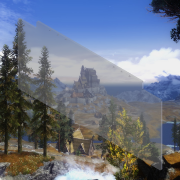
# Autodesk Inventor part: C17_TK_VerticalElectricBoard
Saved by Autodesk Inventor 2015 SP1 (Build 190203100, 203)
## iProperties
Created: 2016-01-21
Part Number: C17_TK_VerticalElectricBoard
Material: Polycarbonate, Clear
Document SubType Name: Modeling
Designer: TheeTimatahee
Density: 1.2 g/cm^3
Appearance: Polycarbonate - Clear
Mass: 547.475 g
Surface Area: 1990.05 cm^2
Volume: 456.229 cm^3
Author: TheeTimatahee
Autodesk Inventor part; units mm, degrees
ref_plane "YZ Plane" through (0, 0, 0) normal (1, 0, 0) x (0, 1, 0)
ref_plane "XZ Plane" through (0, 0, 0) normal (0, 1, 0) x (-1, 0, 0)
ref_plane "XY Plane" through (0, 0, 0) normal (0, 0, 1) x (1, 0, 0)
sketch "Sketch1" plane through (0, 0, 0) normal (0, 0, 1) x (1, 0, 0)
  line L0 (-228.6, -107.95) -> (228.6, -107.95)
  line L1 (168.402, 107.95) -> (-168.402, 107.95)
  line L2 (-171.577, 91.059) -> (-171.577, 109.9058) projected
  line L3 (-171.577, 91.059) -> (-173.736, 88.9) projected
  line L4 (-232.664, 88.9) -> (-173.736, 88.9) projected
  line L5 (-232.664, 88.9) -> (-234.823, 91.059) projected
  line L6 (-234.823, 109.9058) -> (-234.823, 91.059) projected
  line L7 (-171.577, 109.9058) -> (-234.823, 109.9058) projected
  circle A0 centre (-177.8, 101.6) radius 2.0701 projected
  circle A1 centre (-190.5, 101.6) radius 2.0701 projected
  circle A2 centre (-203.2, 101.6) radius 2.0701 projected
  circle A3 centre (-215.9, 101.6) radius 2.0701 projected
  circle A4 centre (-228.6, 101.6) radius 2.0701 projected
  line L8 (234.823, 109.9058) -> (234.823, 91.059) projected
  line L9 (234.823, 91.059) -> (232.664, 88.9) projected
  line L10 (173.736, 88.9) -> (232.664, 88.9) projected
  line L11 (173.736, 88.9) -> (171.577, 91.059) projected
  line L12 (171.577, 109.9058) -> (171.577, 91.059) projected
  line L13 (234.823, 109.9058) -> (171.577, 109.9058) projected
  circle A5 centre (177.8, 101.6) radius 2.0701 projected
  circle A6 centre (190.5, 101.6) radius 2.0701 projected
  circle A7 centre (203.2, 101.6) radius 2.0701 projected
  circle A8 centre (215.9, 101.6) radius 2.0701 projected
  circle A9 centre (228.6, 101.6) radius 2.0701 projected
  line L14 (168.402, 107.95) -> (168.402, 85.725)
  line L15 (168.402, 85.725) -> (228.6, 85.725)
  line L16 (-168.402, 107.95) -> (-168.402, 85.725)
  line L17 (-168.402, 85.725) -> (-228.6, 85.725)
  line L18 (-228.6, 85.725) -> (-228.6, -107.95)
  line L19 (228.6, -107.95) -> (228.6, 85.725)
  point P0 (0, 0)
  dimension "d4" = 3.175
  dimension "d5" = 3.175
  dimension "d6" = 3.175
  dimension "d7" = 3.175
  dimension "d8" = 457.2
  dimension "d9" = 215.9
  constraints: 16 end point, 2 parallel, 1 horizontal, 1 perpendicular
  measures "d4" distance between parallel lines of L10 L15
  measures "d5" distance between parallel lines of L12 L14
  measures "d6" distance between parallel lines of L4 L17
  measures "d7" distance between parallel lines of L16 L2
  measures "d8" distance of L0.start L0.end
  measures "d9" distance between parallel lines of L1 L0
extrude "Extrusion1" add sketch "Sketch1" along normal blind 4.7625 contours L18 L17 L16 L1 L14 L15 L19 L0
fillet "Fillet1" radius 3.175 8 edges at (228.6, -107.95, 2.3813) (168.402, 107.95, 2.3813) (168.402, 85.725, 2.3813) (228.6, 85.725, 2.3813) (-168.402, 107.95, 2.3813) (-168.402, 85.725, 2.3813) (-228.6, 85.725, 2.3813) (-228.6, -107.95, 2.3813)
sketch "Sketch2" plane through (0, 0, 0) normal (0, 0, -1) x (-1, 0, 0)
  arc A0 (103.6687, -25.2476) -> (99.5313, -25.2476) centre (101.6, -25.3238) ccw projected
  line L0 (78.2687, -25.2476) -> (99.5313, -25.2476) projected
  arc A1 (78.2687, -25.2476) -> (74.1313, -25.2476) centre (76.2, -25.3238) ccw projected
  line L1 (52.8687, -25.2476) -> (74.1313, -25.2476) projected
  arc A2 (52.8687, -25.2476) -> (48.7313, -25.2476) centre (50.8, -25.3238) ccw projected
  line L2 (27.4687, -25.2476) -> (48.7313, -25.2476) projected
  arc A3 (27.4687, -25.2476) -> (23.3313, -25.2476) centre (25.4, -25.3238) ccw projected
  line L3 (2.0687, -25.2476) -> (23.3313, -25.2476) projected
  arc A4 (2.0687, -25.2476) -> (-2.0687, -25.2476) centre (0, -25.3238) ccw projected
  line L4 (-23.3313, -25.2476) -> (-2.0687, -25.2476) projected
  arc A5 (-23.3313, -25.2476) -> (-27.4687, -25.2476) centre (-25.4, -25.3238) ccw projected
  line L5 (-48.7313, -25.2476) -> (-27.4687, -25.2476) projected
  arc A6 (-48.7313, -25.2476) -> (-52.8687, -25.2476) centre (-50.8, -25.3238) ccw projected
  line L6 (-74.1313, -25.2476) -> (-52.8687, -25.2476) projected
  arc A7 (-74.1313, -25.2476) -> (-78.2687, -25.2476) centre (-76.2, -25.3238) ccw projected
  line L7 (-99.5313, -25.2476) -> (-78.2687, -25.2476) projected
  arc A8 (-99.5313, -25.2476) -> (-103.6687, -25.2476) centre (-101.6, -25.3238) ccw projected
  line L8 (-124.9313, -25.2476) -> (-103.6687, -25.2476) projected
  arc A9 (-124.9313, -25.2476) -> (-129.0687, -25.2476) centre (-127, -25.3238) ccw projected
  line L9 (-355.6, -25.2476) -> (-129.0687, -25.2476) projected
  line L10 (-355.6, -12.6238) -> (-355.6, -25.2476) projected
  line L11 (355.6, -12.6238) -> (-355.6, -12.6238) projected
  line L12 (355.6, -25.2476) -> (355.6, -12.6238) projected
  line L13 (129.0687, -25.2476) -> (355.6, -25.2476) projected
  arc A10 (129.0687, -25.2476) -> (124.9313, -25.2476) centre (127, -25.3238) ccw projected
  line L14 (103.6687, -25.2476) -> (124.9313, -25.2476) projected
  arc A11 (-99.5313, 101.7524) -> (-103.6687, 101.7524) centre (-101.6, 101.6762) ccw projected
  line L15 (-124.9313, 101.7524) -> (-103.6687, 101.7524) projected
  arc A12 (-124.9313, 101.7524) -> (-129.0687, 101.7524) centre (-127, 101.6762) ccw projected
  line L16 (-175.7355, 101.7524) -> (-129.0687, 101.7524) projected
  arc A13 (-175.7355, 101.7524) -> (-179.8645, 101.7524) centre (-177.8, 101.6) ccw projected
  line L17 (-188.4355, 101.7524) -> (-179.8645, 101.7524) projected
  arc A14 (-188.4355, 101.7524) -> (-192.5645, 101.7524) centre (-190.5, 101.6) ccw projected
  line L18 (-201.1355, 101.7524) -> (-192.5645, 101.7524) projected
  arc A15 (-201.1355, 101.7524) -> (-205.2645, 101.7524) centre (-203.2, 101.6) ccw projected
  line L19 (-213.8355, 101.7524) -> (-205.2645, 101.7524) projected
  arc A16 (-213.8355, 101.7524) -> (-217.9645, 101.7524) centre (-215.9, 101.6) ccw projected
  line L20 (-226.5355, 101.7524) -> (-217.9645, 101.7524) projected
  arc A17 (-226.5355, 101.7524) -> (-230.6645, 101.7524) centre (-228.6, 101.6) ccw projected
  line L21 (-355.6, 101.7524) -> (-230.6645, 101.7524) projected
  line L22 (-355.6, 114.3) -> (-355.6, 101.7524) projected
  line L23 (355.6, 114.3) -> (-355.6, 114.3) projected
  line L24 (355.6, 101.7524) -> (355.6, 114.3) projected
  line L25 (230.6645, 101.7524) -> (355.6, 101.7524) projected
  arc A18 (230.6645, 101.7524) -> (226.5355, 101.7524) centre (228.6, 101.6) ccw projected
  line L26 (217.9645, 101.7524) -> (226.5355, 101.7524) projected
  arc A19 (217.9645, 101.7524) -> (213.8355, 101.7524) centre (215.9, 101.6) ccw projected
  line L27 (205.2645, 101.7524) -> (213.8355, 101.7524) projected
  arc A20 (205.2645, 101.7524) -> (201.1355, 101.7524) centre (203.2, 101.6) ccw projected
  line L28 (192.5645, 101.7524) -> (201.1355, 101.7524) projected
  arc A21 (192.5645, 101.7524) -> (188.4355, 101.7524) centre (190.5, 101.6) ccw projected
  line L29 (179.8645, 101.7524) -> (188.4355, 101.7524) projected
  arc A22 (179.8645, 101.7524) -> (175.7355, 101.7524) centre (177.8, 101.6) ccw projected
  line L30 (129.0687, 101.7524) -> (175.7355, 101.7524) projected
  arc A23 (129.0687, 101.7524) -> (124.9313, 101.7524) centre (127, 101.6762) ccw projected
  line L31 (103.6687, 101.7524) -> (124.9313, 101.7524) projected
  arc A24 (103.6687, 101.7524) -> (99.5313, 101.7524) centre (101.6, 101.6762) ccw projected
  line L32 (78.2687, 101.7524) -> (99.5313, 101.7524) projected
  arc A25 (78.2687, 101.7524) -> (74.1313, 101.7524) centre (76.2, 101.6762) ccw projected
  line L33 (64.0989, 101.7524) -> (74.1313, 101.7524) projected
  spline S0 degree 2 poles (64.0989, 101.7524) (63.534, 102.6488) (62.8722, 103.4567) knots 1.72164 1.72164 1.72164 2 2 2 projected
  spline S1 degree 2 poles (62.8722, 103.4567) (60.4022, 106.3898) (53.1156, 109.5391) (47.8051, 109.5391) knots 0 0 0 1 2 2 2 projected
  spline S2 degree 2 poles (47.8051, 109.5391) (46.0143, 109.5391) (42.1241, 109.076) (41.4757, 108.8907) knots 0 0 0 1 2 2 2 projected
  line L34 (41.4757, 108.8907) -> (41.4757, 101.7524) projected
  line L35 (33.0922, 101.7524) -> (41.4757, 101.7524) projected
  spline S3 degree 2 poles (33.0922, 101.7524) (32.0797, 104.0718) (30.2062, 105.7723) knots 1.066482 1.066482 1.066482 2 2 2 projected
  spline S4 degree 2 poles (30.2062, 105.7723) (28.1994, 107.5939) (22.7036, 109.6008) (18.6898, 109.6008) knots 0 0 0 1 2 2 2 projected
  spline S5 degree 2 poles (18.6898, 109.6008) (14.429, 109.57) (8.3157, 108.1806) (6.3088, 107.2852) knots 0 0 0 1 2 2 2 projected
  line L36 (6.3088, 107.2852) -> (6.3088, 101.7524) projected
  line L37 (-0.2839, 101.7524) -> (6.3088, 101.7524) projected
  spline S6 degree 2 poles (-0.2839, 101.7524) (-1.2964, 104.0718) (-3.1699, 105.7723) knots 1.066482 1.066482 1.066482 2 2 2 projected
  spline S7 degree 2 poles (-3.1699, 105.7723) (-5.1767, 107.5939) (-10.6725, 109.6008) (-14.6863, 109.6008) knots 0 0 0 1 2 2 2 projected
  spline S8 degree 2 poles (-14.6863, 109.6008) (-18.9471, 109.57) (-25.0604, 108.1806) (-27.0673, 107.2852) knots 0 0 0 1 2 2 2 projected
  line L38 (-27.0673, 107.2852) -> (-27.0673, 101.7524) projected
  line L39 (-41.1772, 101.7524) -> (-27.0673, 101.7524) projected
  line L40 (-41.1772, 101.7524) -> (-41.1772, 102.1599) projected
  line L41 (-41.1772, 102.1599) -> (-33.3349, 102.1599) projected
  line L42 (-33.3349, 102.1599) -> (-33.3349, 108.7981) projected
  line L43 (-33.3349, 108.7981) -> (-58.4982, 108.7981) projected
  line L44 (-58.4982, 108.7981) -> (-58.4982, 102.1599) projected
  line L45 (-58.4982, 102.1599) -> (-50.4707, 102.1599) projected
  line L46 (-50.4707, 102.1599) -> (-50.4707, 101.7524) projected
  line L47 (-74.1313, 101.7524) -> (-50.4707, 101.7524) projected
  arc A26 (-74.1313, 101.7524) -> (-78.2687, 101.7524) centre (-76.2, 101.6762) ccw projected
  line L48 (-99.5313, 101.7524) -> (-78.2687, 101.7524) projected
  point P0 (0, 0)
hole "Hole1" at (-127, 101.6762, 0) at (-101.6, 101.6762, 0) at (-76.2, 101.6762, 0) at (76.2, 101.6762, 0) at (101.6, 101.6762, 0) at (127, 101.6762, 0) at (-127, -25.3238, 0) at (-101.6, -25.3238, 0) at (-76.2, -25.3238, 0) at (-50.8, -25.3238, 0) at (-25.4, -25.3238, 0) at (0, -25.3238, 0) at (25.4, -25.3238, 0) at (50.8, -25.3238, 0) at (76.2, -25.3238, 0) at (101.6, -25.3238, 0) at (127, -25.3238, 0) direction (0, 0, 1) diameter 4.1402 end through all
sketch "Sketch4" plane through (0, 0, 0) normal (0, 0, -1) x (-1, 0, 0)
  line L0 (-165.227, 107.95) -> (165.227, 107.95) projected
  line L1 (107.95, -107.95) -> (-107.95, -107.95) construction
  line L2 (-107.95, -107.95) -> (-107.95, 107.95) construction
  line L3 (-107.95, 107.95) -> (107.95, 107.95) construction
  line L4 (107.95, 107.95) -> (107.95, -107.95) construction
  line L5 (197.0019, -39.6304) -> (129.4704, -39.6304) construction
  line L6 (129.4704, -39.6304) -> (129.4704, 38.94) construction
  line L7 (129.4704, 38.94) -> (197.0019, 38.94) construction
  line L8 (197.0019, 38.94) -> (197.0019, -39.6304) construction
  line L9 (-125.3858, -27.2271) -> (-180.4191, -27.2271) construction
  line L10 (-180.4191, -27.2271) -> (-180.4191, 36.8021) construction
  line L11 (-180.4191, 36.8021) -> (-125.3858, 36.8021) construction
  line L12 (-125.3858, 36.8021) -> (-125.3858, -27.2271) construction
  line L13 (-51.4537, 12.8385) -> (-125.3858, 12.8385) construction
  line L14 (-125.3858, 12.8385) -> (-125.3858, -68.9649) construction
  line L15 (-125.3858, -68.9649) -> (-51.4537, -68.9649) construction
  line L16 (-51.4537, -68.9649) -> (-51.4537, 12.8385) construction
  line L17 (225.425, -107.95) -> (-225.425, -107.95) projected
  line L18 (-228.6, -104.775) -> (-228.6, 82.55) projected
  point P0 (0, 0)
  constraints: 2 collinear, 8 other
decal "Decal1"
decal "Decal2"
decal "Decal3"
body "Solid1"
